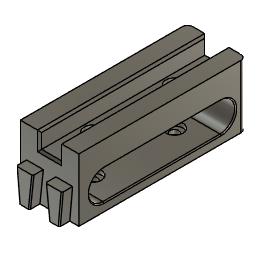
Slider_bottom (Autodesk Fusion 360 design; units mm, degrees)
Autodesk Fusion 360 part; units mm, degrees
note: some values were not read from the file. Chosen so that the rebuilt part matches the saved one: which bodies a step acts on.
sketch "Sketch1" plane through (0, 0, 0) normal (0, 1, 0) x (1, 0, 0)
  line L0 (0, 0) -> (28, 0)
  line L1 (28, 0) -> (28, -30)
  line L2 (0, 0) -> (0, -30)
  line L3 (0, -30) -> (9.2, -30)
  line L4 (28, -30) -> (18.8, -30)
  line L5 (18.8, -30) -> (18.8, -22)
  line L6 (9.2, -30) -> (9.2, -22)
  line L7 (9.2, -22) -> (18.8, -22)
  dimension "d1" = 28
  dimension "d2" = 30
  dimension "d3" = 30
  dimension "d4" = 9.2
  dimension "d5" = 9.2
  dimension "d6" = 8
  dimension "d7" = 8
  dimension "d53" = 9.6
  constraint coincident L0.start L2.start
  constraint horizontal L0
  constraint perpendicular L0 L1
  constraint perpendicular L0 L2
  constraint perpendicular L2 L3
  constraint perpendicular L1 L4
  constraint perpendicular L4 L5
  constraint perpendicular L3 L6
  measures "d1" distance of L0.start L0.end
  measures "d2" distance of L0.end L1.end
  measures "d3" distance of L0.start L2.end
  measures "d4" distance of L2.end L3.end
  measures "d5" distance of L1.end L4.end
  measures "d6" distance of L4.end L5.end L0.start
  measures "d7" distance of L3.end L6.end L0.start
  measures "d31" distance of L0.start
  measures "d53" distance of L5.end L6.end L0.start
extrude "Extrude1" add sketch "Sketch1" along normal blind 80 makes body 1
sketch "Sketch2" plane through (0, 0, 0) normal (-1, 0, 0) x (0, -1, 0)
  line L0 (0, 0) -> (0, 30)
  line L1 (0, 30) -> (-80, 30)
  line L2 (-80, 30) -> (-80, 0)
  line L3 (-80, 0) -> (0, 0)
  line L4 (0, 0) -> (-80, 0)
  line L5 (-80, 0) -> (-80, 22)
  line L6 (-80, 22) -> (0, 22)
  line L7 (0, 22) -> (0, 0)
  line L8 (0, 22) -> (-80, 0) construction
  line L9 (-80, 22) -> (0, 0) construction
  line L10 (-5, 17) -> (-5, 5) construction
  line L11 (-75, 5) -> (-75, 17) construction
  line L12 (-75, 11) -> (-68, 11) construction
  line L13 (-5, 11) -> (-12, 11) construction
  line L14 (-68, 4) -> (-12, 4)
  arc A0 (-12, 4) -> (-12, 18) centre (-12, 11) ccw
  line L15 (-12, 18) -> (-68, 18)
  arc A1 (-68, 18) -> (-68, 4) centre (-68, 11) ccw
  line L16 (-68, 11) -> (-12, 11) construction
  dimension "d10" = 80
  dimension "d11" = 22
  dimension "d13" = 5
  dimension "d14" = 5
  dimension "d15" = 7
  dimension "d16" = 7
  dimension "d17" = 14
  constraint horizontal L4
  constraint vertical L5
  constraint horizontal L6
  constraint vertical L7
  constraint coincident L0.start L3.end
  constraint parallel L7 L10
  constraint parallel L5 L11
  constraint midpoint L11 L12.start
  constraint perpendicular L11 L12
  constraint midpoint L10 L13.start
  constraint perpendicular L10 L13
  constraint tangent L14 A0
  constraint tangent A0 L15
  constraint parallel L14 L15
  constraint tangent L15 A1
  constraint tangent L14 A1
  constraint coincident L13.end A0.centre
  constraint parallel L13 L16
  constraint coincident L12.end A1.centre
  measures "d10" distance of L0.start L2.end
  measures "d11" distance of L0.start L6.end
  measures "d13" distance of L5 L11
  measures "d14" distance of L7 L10
  measures "d15" distance of L12.start L12.end
  measures "d16" distance of L13.start L13.end
  measures "d17" diameter of A0
extrude "Extrude2" cut sketch "Sketch2" against normal up to surface (28 mm away) contours L14 A0 L15 A1 bodies 1
chamfer "Chamfer1" distance 1 angle 45 8 edges at (9.2, 0, 26) (14, 0, 22) (18.8, 0, 26) (9.2, 80, 26) (14, 80, 22) (18.8, 80, 26) (18.8, 40, 30) (9.2, 40, 30) on bodies 1
fillet "Fillet1" radius 0.5 8 edges at (28, 40, 4) (28, 5, 11) (28, 40, 18) (28, 75, 11) (0, 40, 4) (0, 75, 11) (0, 40, 18) (0, 5, 11) on bodies 1
sketch "Sketch3" plane through (0, 0, 22) normal (0, 0, 1) x (-1, 0, 0)
  line L0 (-9.2, -79) -> (-9.2, -1)
  line L1 (-18.8, -1) -> (-18.8, -79)
  line L2 (-9.2, -68) -> (-19.2, -68)
  line L3 (-19.2, -68) -> (-19.2, -12)
  line L4 (-19.2, -12) -> (-9.2, -12)
  line L5 (-9.2, -12) -> (-9.2, -68)
  line L6 (-14, -79) -> (-14.2, -68) construction
  line L7 (-14.2, -12) -> (-14, -1) construction
  line L8 (-14.2, -68) -> (-14.2, -12) construction
  circle A0 centre (-14.2, -20.5) radius 2.1
  circle A1 centre (-14.2, -59.5) radius 2.1
  line L9 (-0.5, -68) -> (-0.5, -12)
  line L10 (-0.5, -12) -> (-27.5, -12)
  line L11 (-27.5, -12) -> (-27.5, -68)
  line L12 (-27.5, -68) -> (-0.5, -68)
  circle A2 centre (-14.2, -59.5) radius 4.1
  circle A3 centre (-14.2, -20.5) radius 4.1
  line L13 (-18.8, -79) -> (-9.2, -79)
  line L14 (-9.2, -1) -> (-18.8, -1)
  dimension "d22" = 10
  dimension "d23" = 56
  dimension "d24" = 4.2
  dimension "d25" = 4.2
  dimension "d30" = 2
  dimension "d31" = 2
  constraint horizontal L2
  constraint vertical L3
  constraint horizontal L4
  constraint vertical L5
  constraint coincident L0 L2.start
  constraint midpoint L2 L6.end
  constraint midpoint L4 L7.start
  constraint equal L6 L7
  constraint coincident L8 A0.centre
  constraint coincident L8 A1.centre
  measures "d22" distance of L2.start L2.end
  measures "d23" distance of L2.start L4.end
  measures "d24" diameter of A0
  measures "d25" diameter of A1
extrude "Extrude4" cut sketch "Sketch3" against normal blind 20 contours A2 | A3 bodies 1 makes body 2 at (16.2584, 59.9161, 20.6667) makes body 3 at (9.3333, 26.6667, 0)
extrude "Extrude3" cut sketch "Sketch3" against normal blind 22 contours A0 | A1 bodies 1 2 3
sketch "Sketch6" plane through (0, 0, 0) normal (0, -1, 0) x (1, 0, 0)
  line L0 (8.2, 30) -> (0, 30)
  line L1 (0, 30) -> (0, 0)
  line L2 (0, 0) -> (28, 0)
  line L3 (28, 0) -> (28, 30)
  line L4 (28, 30) -> (19.8, 30)
  line L5 (0, 0) -> (14, 0)
  line L6 (14, 0) -> (14, 21)
  line L7 (14, 21) -> (0, 21)
  line L8 (0, 21) -> (0, 0)
  line L9 (14, 21) -> (28, 21)
  line L10 (28, 21) -> (28, 0)
  line L11 (28, 0) -> (14, 0)
  line L12 (14, 0) -> (14, 21)
  line L13 (7, 0) -> (7, 21) construction
  line L14 (3, 15) -> (7, 15)
  line L15 (7, 15) -> (11, 15)
  line L16 (3, 15) -> (4.3621, 0)
  line L17 (11, 15) -> (9.3621, 0)
  line L18 (9.3621, 0) -> (4.3621, 0)
  line L19 (25, 15) -> (23.6379, 0)
  line L20 (17, 15) -> (18.6379, 0)
  line L21 (21, 15) -> (17, 15)
  line L22 (25, 15) -> (21, 15)
  line L23 (18.6379, 0) -> (23.6379, 0)
  line L24 (19.8, 30) -> (19.8, 21)
  line L25 (19.8, 21) -> (8.2, 21)
  line L26 (8.2, 21) -> (8.2, 30)
  dimension "d47" = 4
  dimension "d48" = 15
  dimension "d49" = 5
  constraint horizontal L5
  constraint vertical L6
  constraint horizontal L7
  constraint vertical L8
  constraint coincident L1.end L2.start
  constraint horizontal L9
  constraint vertical L10
  constraint horizontal L11
  constraint vertical L12
  constraint coincident L2.end L3.start
  constraint midpoint L5 L13.start
  constraint midpoint L7 L13.end
  constraint coincident L13 L14.end
  constraint perpendicular L13 L14
  constraint perpendicular L13 L15
  constraint equal L14 L15
  constraint coincident L2 L16.end
  constraint coincident L2 L17.end
  constraint symmetric L12 L14.start L19.start
  constraint symmetric L12 L14.end L21.start
  constraint symmetric L12 L15.end L20.start
  constraint symmetric L12 L16.end L19.end
  constraint symmetric L12 L17.end L20.end
  measures "d47" distance of L14.end L15.end
  measures "d48" distance of L5 L14
  measures "d49" distance of L16.end L17.end
extrude "Extrude5" add sketch "Sketch6" along normal blind 5 contours L2 L5 L14 L15 L16 L17 L18 | L2 L11 L19 L20 L21 L22 L23 bodies 1 2 3
chamfer "Chamfer3" distance 0.5 angle 45 4 edges at (24.319, -5, 7.5) (17.819, -5, 7.5) (10.181, -5, 7.5) (3.681, -5, 7.5) on bodies 1
fillet "Fillet2" radius 2.5 2 edges at (28, 80, 15) (0, 80, 15) on bodies 1
